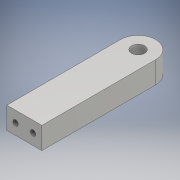
# Autodesk Inventor part: SupportCylinder
Saved by Autodesk Inventor 2018 (Build 220112000, 112)
## iProperties
Created: 2019-05-10
Part Number: SupportCylinder
Material: Generic
Document SubType Name: Modeling
Designer: aal_9
Density: 1 g/cm^3
Appearance: Default
Author: aal_9
Autodesk Inventor part; units mm, degrees
ref_plane "YZ Plane" through (0, 0, 0) normal (1, 0, 0) x (0, 1, 0)
ref_plane "XZ Plane" through (0, 0, 0) normal (0, 1, 0) x (-1, 0, 0)
ref_plane "XY Plane" through (0, 0, 0) normal (0, 0, 1) x (1, 0, 0)
sketch "Sketch1" plane through (0, 0, 0) normal (0, 0, 1) x (1, 0, 0)
  line L0 (0, 0) -> (16, 0)
  line L1 (16, 0) -> (16, 60)
  line L2 (16, 60) -> (0, 60)
  line L3 (0, 60) -> (0, 0)
  circle A0 centre (8, 52) radius 3
  dimension "d9" = 16
  dimension "d10" = 60
  dimension "d11" = 6
  dimension "d12" = 8
  constraints: 8 end point, 2 parallel, 1 centre point, 1 horizontal, 1 perpendicular
  measures "d9" distance of L2.end L1.end
  measures "d10" distance of L1.end L0.end
  measures "d11" diameter of A0
  measures "d12" distance from line of L2 A0.centre
extrude "Extrusion1" add sketch "Sketch1" along normal blind 10
sketch "Sketch2" plane through (0, 0, 10) normal (0, 0, 1) x (1, 0, 0)
  line L0 (16, 60) -> (0, 60) projected
  circle A0 centre (8, 52) radius 3 projected
  arc A1 (16, 52) -> (0, 52) centre (8, 52) ccw
  line L1 (16.7201, 52) -> (16.7201, 60.3787)
  line L2 (16.7201, 60.3787) -> (-0.5009, 60.3787)
  line L3 (-0.5009, 60.3787) -> (-0.5009, 52)
  line L4 (-0.5009, 52) -> (0, 52)
  line L5 (16, 52) -> (16.7201, 52)
  point P0 (0, 0)
  constraints: 10 end point, 3 parallel, 2 horizontal, 2 perpendicular, 2 point on circle, 1 centre point, 1 coincident
extrude "Extrusion2" cut sketch "Sketch2" against normal up to next contours A1 L4 L3 L2 L1 L5
sketch "Sketch3" plane through (0, 0, 0) normal (0, -1, 0) x (1, 0, 0)
  line L0 (0, 10) -> (16, 10) projected
  line L1 (0, 0) -> (16, 0) projected
  line L2 (0, 0) -> (0, 10) projected
  line L3 (16, 0) -> (16, 10) projected
  point P0 (4, 5)
  point P1 (12, 5)
  dimension "d19" = 5
  dimension "d20" = 5
  dimension "d21" = 4
  dimension "d22" = 4
  measures "d19" distance from line of L0 point (4, 5)
  measures "d20" distance from line of L1 point (12, 5)
  measures "d21" distance from line of L2 point (4, 5)
  measures "d22" distance from line of L3 point (12, 5)
hole "Hole1" at (4, 0, 5) at (12, 0, 5) direction (0, 1, 0) diameter 2.459 depth 8.8 tip angle 118 thread size "M3x0.5" class "6H" standard "ANSI Metric M Profile"
body "Solid1"
